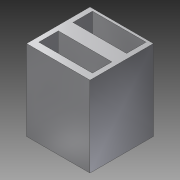
# Autodesk Inventor part: USB
Saved by Autodesk Inventor 2015 (Build 190159000, 159)
## iProperties
Created: 2015-12-03
Part Number: USB
Material: Generic
Document SubType Name: Modeling
Designer: david
Density: 1 g/cm^3
Appearance: Aluminum - Polished
Author: david
Autodesk Inventor part; units mm, degrees
ref_plane "YZ Plane" through (0, 0, 0) normal (1, 0, 0) x (0, 1, 0)
ref_plane "XZ Plane" through (0, 0, 0) normal (0, 1, 0) x (-1, 0, 0)
ref_plane "XY Plane" through (0, 0, 0) normal (0, 0, 1) x (1, 0, 0)
sketch "Sketch1" plane through (0, 0, 0) normal (0, 1, 0) x (-1, 0, 0)
  line L0 (-6.5, 8.25) -> (6.5, 8.25)
  line L1 (6.5, 8.25) -> (6.5, -8.25)
  line L2 (6.5, -8.25) -> (-6.5, -8.25)
  line L3 (-6.5, -8.25) -> (-6.5, 8.25)
  line L4 (-6.5, 8.25) -> (6.5, -8.25) construction
  line L5 (6.5, 8.25) -> (-6.5, -8.25) construction
  point P0 (0, 0)
  dimension "d0" = 13
  dimension "d1" = 16.5
  constraints: 12 end point, 2 midpoint, 2 parallel, 1 horizontal, 1 perpendicular
  measures "d0" distance of L1.end L2.end
  measures "d1" distance of L0.end L1.end
extrude "Extrusion1" add sketch "Sketch1" along normal blind 13
sketch "Sketch2" plane through (-6.5, 0, 8.25) normal (0, 0, 1) x (1, 0, 0)
  line L0 (1, 8.5) -> (12, 8.5)
  line L1 (12, 8.5) -> (12, 12.5)
  line L2 (12, 12.5) -> (1, 12.5)
  line L3 (1, 12.5) -> (1, 8.5)
  line L4 (0, 13) -> (13, 13) projected
  line L5 (0, 0) -> (0, 13) projected
  line L6 (1, 5.5) -> (12, 5.5)
  line L7 (12, 5.5) -> (12, 1.5)
  line L8 (12, 1.5) -> (1, 1.5)
  line L9 (1, 1.5) -> (1, 5.5)
  point P0 (6.5, 0)
  dimension "d4" = 11
  dimension "d5" = 4
  dimension "d6" = 0.5
  dimension "d7" = 1
  dimension "d8" = 11
  dimension "d9" = 4
  dimension "d10" = 3
  dimension "d11" = 1
  constraints: 16 end point, 4 parallel, 2 horizontal, 2 perpendicular
  measures "d4" distance of L2.end L1.end
  measures "d5" distance of L1.end L0.end
  measures "d6" distance between parallel lines of L4 L2
  measures "d7" distance between parallel lines of L5 L3
  measures "d8" distance of L7.end L8.end
  measures "d9" distance of L6.end L7.end
  measures "d10" distance between parallel lines of L0 L6
  measures "d11" distance between parallel lines of L5 L9
extrude "Extrusion2" cut sketch "Sketch2" against normal blind 13
body "Solid1"
